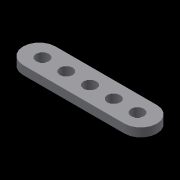
# Autodesk Inventor part: ShinExtender
Saved by Autodesk Inventor 2015 SP1 (Build 190203100, 203)
## iProperties
Created: 2015-05-16
Part Number: ShinExtender
Material: Generic
Document SubType Name: Modeling
Designer: Val
Density: 1 g/cm^3
Appearance: Default
Author: Val
Autodesk Inventor part; units mm, degrees
ref_plane "YZ Plane" through (0, 0, 0) normal (1, 0, 0) x (0, 1, 0)
ref_plane "XZ Plane" through (0, 0, 0) normal (0, 1, 0) x (-1, 0, 0)
ref_plane "XY Plane" through (0, 0, 0) normal (0, 0, 1) x (1, 0, 0)
sketch "Base" plane through (0, 0, 0) normal (0, 0, 1) x (1, 0, 0)
  circle A0 centre (0, 0) radius 3
  line L0 (0, 0) -> (-11, 0) construction
  circle A1 centre (-11, 0) radius 3
  line L1 (0, 0) -> (11, 0) construction
  circle A2 centre (11, 0) radius 3
  line L2 (11, 0) -> (22, 0) construction
  circle A3 centre (22, 0) radius 3
  line L3 (-11, 0) -> (-22, 0) construction
  circle A4 centre (-22, 0) radius 3
  line L4 (-23.5, 7.5) -> (23.5, 7.5)
  line L5 (-23.5, -7.5) -> (23.5, -7.5)
  arc A5 (-23.5, 7.5) -> (-23.5, -7.5) centre (-23.5, 0) ccw
  arc A6 (23.5, -7.5) -> (23.5, 7.5) centre (23.5, 0) ccw
  dimension "d0" = 6
  dimension "d1" = 11
  dimension "d4" = 7.5
  dimension "d5" = 7.5
  dimension "d6" = 1.5
  dimension "d7" = 1.5
  constraints: 12 end point, 7 centre point, 6 horizontal, 5 coincident, 4 equal radius, 4 point on circle, 4 tangent, 3 collinear
  measures "d0" diameter of A0
  measures "d1" distance of L0.start L0.end
  measures "d4" distance between parallel lines of L4 L0
  measures "d5" distance between parallel lines of L5 L0
  measures "d6" distance of L3.end A5.centre
  measures "d7" distance of A6.centre L2.end
extrude "BaseFeature" add sketch "Base" along normal blind 4
equation "\"d5\" = d4"
equation "\"d6\" = d4 - d0"
equation "\"d7\" = d6"
